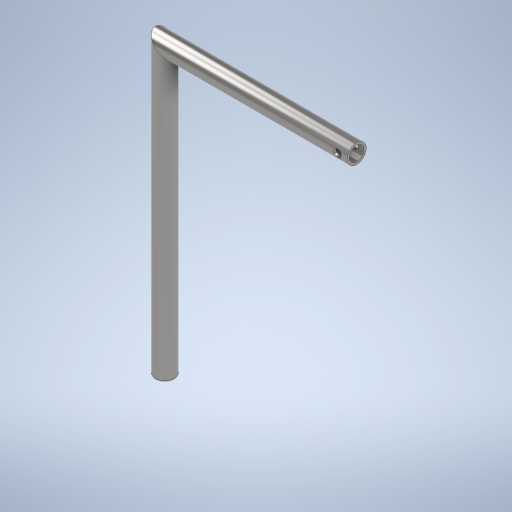
# Autodesk Inventor part: Steuerhebel
Saved by Autodesk Inventor 2024.4 (Build 284460000, 460)
## iProperties
Created: 2026-01-20
Part Number: Steuerhebel
Material: Edelstahl
Document SubType Name: Modeling
Designer: Philf
Density: 8 g/cm^3
Appearance: Halbpoliert
Description: Steuerhebel
Mass: 68.4618 g
Surface Area: 551.776 cm^2
Volume: 68.4618 cm^3
Masse[kg]: 0,0000 kg
Autodesk Inventor part; units mm, degrees
ref_plane "YZ Plane" through (0, 0, 0) normal (1, 0, 0) x (0, 1, 0)
ref_plane "XZ Plane" through (0, 0, 0) normal (0, 1, 0) x (-1, 0, 0)
ref_plane "XY Plane" through (0, 0, 0) normal (0, 0, 1) x (1, 0, 0)
sketch "Skizze12" plane through (0, 0, 0) normal (0, 1, 0) x (-1, 0, 0)
  line L0 (0, 0) -> (200, 0)
  line L1 (200, 0) -> (200, -300)
  dimension "d28" = 200
  dimension "d29" = 300
  constraints: 4 end point, 1 horizontal, 1 perpendicular
  measures "d28" distance of L0.start L0.end
  measures "d29" distance of L0.end L1.end
sketch "Skizze13" plane through (0, 0, 0) normal (1, 0, 0) x (0, 1, 0)
  circle A0 centre (0, 0) radius 10
  circle A1 centre (0, 0) radius 7.5
  dimension "d30" = 20
  dimension "d31" = 15
  constraints: 2 centre point, 2 coincident
  measures "d30" diameter of A0
  measures "d31" diameter of A1
sweep "Sweeping2" add profiles "Skizze13" path "Skizze12"
sketch "Skizze14" plane through (0, 0, 0) normal (0, 1, 0) x (-1, 0, 0)
  line L0 (0, 0) -> (10, 0)
  circle A0 centre (10, 0) radius 4
  dimension "d34" = 10
  dimension "d35" = 8
  constraints: 2 end point, 1 centre point, 1 coincident, 1 horizontal
  measures "d34" distance of L0.start L0.end
  measures "d35" diameter of A0
extrude "Extrusion3" cut sketch "Skizze14" along normal through all both and the other way through all
fillet "Rundung1" radius 2 2 edges at (-200, -10, -300) (-200, -7.5, -300)
